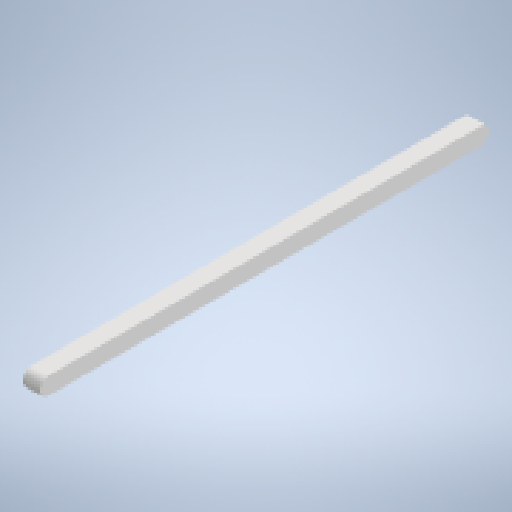
# Autodesk Inventor part: Link 250
Saved by Autodesk Inventor 2023 (Build 270158000, 158)
## iProperties
Created: 2024-01-18
Part Number: Link 250
Material: Generic
Document SubType Name: Modeling
Designer: juanp
Density: 1 g/cm^3
Appearance: Default
Author: juanp
Autodesk Inventor part; units mm, degrees
ref_plane "YZ Plane" through (0, 0, 0) normal (1, 0, 0) x (0, 1, 0)
ref_plane "XZ Plane" through (0, 0, 0) normal (0, 1, 0) x (-1, 0, 0)
ref_plane "XY Plane" through (0, 0, 0) normal (0, 0, 1) x (1, 0, 0)
sketch "Sketch1" plane through (0, 0, 0) normal (1, 0, 0) x (0, 1, 0)
  line L0 (0, -62.5) -> (0, 62.5) construction
  line L1 (5, -62.5) -> (5, 62.5)
  line L2 (-5, 62.5) -> (-5, -62.5)
  arc A0 (-5, -62.5) -> (5, -62.5) centre (0, -62.5) ccw
  arc A1 (5, 62.5) -> (-5, 62.5) centre (0, 62.5) ccw
  point P0 (0, 0)
  dimension "d0" = 125
  dimension "d1" = 10
  constraints: 8 end point, 4 point on circle, 4 tangent, 2 centre point, 1 midpoint, 1 parallel, 1 vertical
  measures "d0" distance of L0.start L0.end
  measures "d1" distance between parallel lines of L1 L2
extrude "Extrusion1" add sketch "Sketch1" along normal blind 10
body "Solid1"
